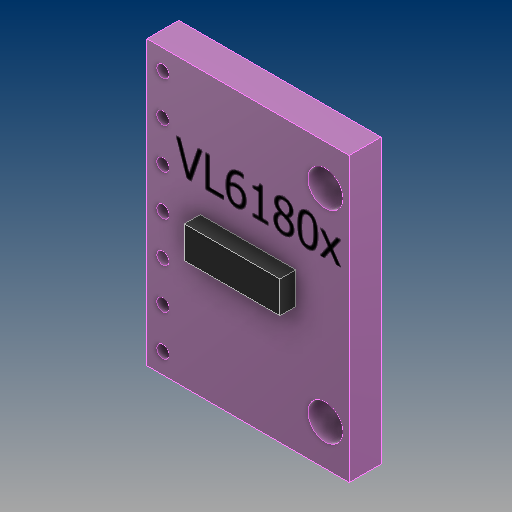
# Autodesk Inventor part: VL6180x_czujnik
Saved by Autodesk Inventor 2021 (Build 250183000, 183)
## iProperties
Created: 2022-05-17
Part Number: VL6180x_czujnik
Material: Generic
Document SubType Name: Modeling
Designer: agnpi
Density: 1 g/cm^3
Appearance: Default
Author: agnpi
Autodesk Inventor part; units mm, degrees
ref_plane "YZ Plane" through (0, 0, 0) normal (1, 0, 0) x (0, 1, 0)
ref_plane "XZ Plane" through (0, 0, 0) normal (0, 1, 0) x (-1, 0, 0)
ref_plane "XY Plane" through (0, 0, 0) normal (0, 0, 1) x (1, 0, 0)
sketch "Sketch1" plane through (0, 0, 0) normal (0, 0, 1) x (1, 0, 0)
  line L0 (-8.89, 0) -> (8.89, 0) projected
  line L1 (0, -12.446) -> (0, 12.446) projected
  line L2 (-6.35, 8.89) -> (6.35, 8.89)
  line L3 (6.35, 8.89) -> (6.35, -8.89)
  line L4 (6.35, -8.89) -> (-6.35, -8.89)
  line L5 (-6.35, -8.89) -> (-6.35, 8.89)
  line L6 (-6.35, 8.89) -> (6.35, -8.89) construction
  line L7 (6.35, 8.89) -> (-6.35, -8.89) construction
  point P0 (0, 0)
  dimension "d0" = 17.78
  dimension "d1" = 12.7
  constraints: 12 end point, 2 midpoint, 2 parallel, 1 horizontal, 1 perpendicular
  measures "d0" distance between parallel lines of L4 L2
  measures "d1" distance between parallel lines of L3 L5
extrude "Extrusion1" add sketch "Sketch1" along normal mid plane 2
sketch "Sketch2" plane through (0, 0, 1) normal (0, 0, 1) x (1, 0, 0)
  line L0 (-6.35, 8.89) -> (-6.35, -8.89) projected
  line L1 (6.35, 8.89) -> (-6.35, 8.89) projected
  line L2 (-6.35, -8.89) -> (6.35, -8.89) projected
  point P0 (0, 0)
  point P1 (-5.35, 0)
  point P2 (-5.35, -2.54)
  point P3 (-5.35, 2.54)
  point P4 (-5.35, -5.08)
  point P5 (-5.35, -7.62)
  point P6 (-5.35, 5.08)
  point P7 (-5.35, 7.62)
  dimension "d11" = 2.54
  dimension "d12" = 1
  dimension "d13" = 1
  dimension "d14" = 1
  dimension "d15" = 1
  dimension "d16" = 2.54
  dimension "d17" = 2.54
  dimension "d18" = 1.27
  dimension "d19" = 1.27
  dimension "d20" = 2.54
  dimension "d21" = 2.54
  dimension "d22" = 1
  dimension "d23" = 1
  dimension "d24" = 1
  measures "d11" distance of point (-5.35, -2.54) point (-5.35, 0)
  measures "d12" distance from line of L0 point (-5.35, 0)
  measures "d13" distance from line of L0 point (-5.35, -2.54)
  measures "d14" distance from line of L0 point (-5.35, -5.08)
  measures "d15" distance from line of L0 point (-5.35, 2.54)
  measures "d16" distance of point (-5.35, 0) point (-5.35, 2.54)
  measures "d17" distance of point (-5.35, -5.08) point (-5.35, -2.54)
  measures "d18" distance from line of L1 point (-5.35, 7.62)
  measures "d19" distance from line of L2 point (-5.35, -7.62)
  measures "d20" distance of point (-5.35, -5.08) point (-5.35, -7.62)
  measures "d21" distance of point (-5.35, 5.08) point (-5.35, 7.62)
  measures "d22" distance from line of L0 point (-5.35, 7.62)
  measures "d23" distance from line of L0 point (-5.35, 5.08)
  measures "d24" distance from line of L0 point (-5.35, -7.62)
hole "Hole1" at (-5.35, 0, 1) at (-5.35, -2.54, 1) at (-5.35, 2.54, 1) at (-5.35, -5.08, 1) at (-5.35, -7.62, 1) at (-5.35, 5.08, 1) at (-5.35, 7.62, 1) direction (0, 0, -1) diameter 0.76 end through all
sketch "Sketch3" plane through (0, 0, 1) normal (0, 0, 1) x (1, 0, 0)
  line L0 (-6.35, -8.89) -> (6.35, -8.89) projected
  line L1 (6.35, -8.89) -> (6.35, 8.89) projected
  point P0 (0, 0)
  point P1 (4.85, 6.35)
  point P2 (4.85, -6.35)
  dimension "d32" = 12.7
  dimension "d33" = 2.54
  dimension "d34" = 1.5
  dimension "d35" = 1.5
  measures "d32" distance of point (4.85, -6.35) point (4.85, 6.35)
  measures "d33" distance from line of L0 point (4.85, -6.35)
  measures "d34" distance from line of L1 point (4.85, 6.35)
  measures "d35" distance from line of L1 point (4.85, -6.35)
hole "Hole2" at (4.85, 6.35, 1) at (4.85, -6.35, 1) direction (0, 0, -1) diameter 2.184 end through all
sketch "Sketch4" plane through (0, 0, 1) normal (0, 0, 1) x (1, 0, 0)
  line L0 (-3, 1) -> (3, 1)
  line L1 (3, 1) -> (3, -1)
  line L2 (3, -1) -> (-3, -1)
  line L3 (-3, -1) -> (-3, 1)
  line L4 (-3, 1) -> (3, -1) construction
  line L5 (3, 1) -> (-3, -1) construction
  point P0 (0, 0)
  dimension "d36" = 6
  dimension "d37" = 2
  constraints: 12 end point, 2 midpoint, 2 parallel, 1 horizontal, 1 perpendicular
  measures "d36" distance of L1.end L2.end
  measures "d37" distance of L0.end L1.end
extrude "Extrusion2" add sketch "Sketch4" along normal blind 1 separate body
sketch "Sketch5" plane through (0, 0, 1) normal (0, 0, 1) x (1, 0, 0)
  line L0 (-4.5172, 4.5869) -> (11.2934, 4.5869) construction
  line L1 (11.2934, 4.5869) -> (11.2934, 1.4006) construction
  line L2 (11.2934, 1.4006) -> (-4.5172, 1.4006) construction
  line L3 (-4.5172, 1.4006) -> (-4.5172, 4.5869) construction
  point P0 (0, 0)
  constraints: 2 other
body "Solid1"
body "Solid2"
